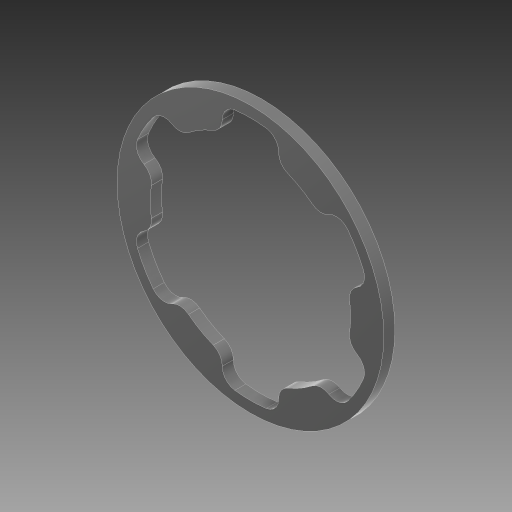
# Autodesk Inventor part: MAXSpline Spacers
Saved by Autodesk Inventor 2023 (Build 270158030, 158C)
## iProperties
Created: 2023-01-27
Part Number: MAXSpline Spacers
Material: Acetal Resin, Black
Document SubType Name: Modeling
Designer: Max Boord
Density: 1.425 g/cm^3
Appearance: Smooth - Black
Author: Max Boord
Mass: 17.9779 g
Surface Area: 108.837 cm^2
Volume: 12.6161 cm^3
Autodesk Inventor part; units mm, degrees
ref_plane "YZ Plane" through (0, 0, 0) normal (1, 0, 0) x (0, 1, 0)
ref_plane "XZ Plane" through (0, 0, 0) normal (0, 1, 0) x (-1, 0, 0)
ref_plane "XY Plane" through (0, 0, 0) normal (0, 0, 1) x (1, 0, 0)
sketch "MAXSpline Spacer Profile" plane through (0, 0, 0) normal (0, 0, 1) x (1, 0, 0)
  circle A0 centre (0, 0) radius 19.05
  arc A1 (15.22, 4.1356) -> (16.1399, 6.7328) centre (14.2452, 5.9424) ccw
  arc A2 (15.22, 4.1356) -> (14.1626, 2.0366) centre (16.1947, 2.3288) ccw
  arc A3 (14.1626, -2.0366) -> (14.1626, 2.0366) centre (0, 0) ccw
  arc A4 (14.1626, -2.0366) -> (15.22, -4.1356) centre (16.1947, -2.3288) ccw
  arc A5 (16.1399, -6.7328) -> (15.22, -4.1356) centre (14.2452, -5.9424) ccw
  arc A6 (13.9007, -10.6112) -> (16.1399, -6.7328) centre (0, 0) ccw
  arc A7 (11.1915, -11.1131) -> (13.9007, -10.6112) centre (12.2689, -9.3655) ccw
  arc A8 (11.1915, -11.1131) -> (8.845, -11.2469) centre (10.1141, -12.8607) ccw
  arc A9 (5.3176, -13.2835) -> (8.845, -11.2469) centre (0, 0) ccw
  arc A10 (5.3176, -13.2835) -> (4.0285, -15.2487) centre (6.0806, -15.1894) ccw
  arc A11 (2.2392, -17.344) -> (4.0285, -15.2487) centre (1.9763, -15.3079) ccw
  arc A12 (-2.2392, -17.344) -> (2.2392, -17.344) centre (0, 0) ccw
  arc A13 (-4.0285, -15.2487) -> (-2.2392, -17.344) centre (-1.9763, -15.3079) ccw
  arc A14 (-4.0285, -15.2487) -> (-5.3176, -13.2835) centre (-6.0806, -15.1894) ccw
  arc A15 (-8.845, -11.2469) -> (-5.3176, -13.2835) centre (0, 0) ccw
  arc A16 (-8.845, -11.2469) -> (-11.1915, -11.1131) centre (-10.1141, -12.8607) ccw
  arc A17 (-13.9007, -10.6112) -> (-11.1915, -11.1131) centre (-12.2689, -9.3655) ccw
  arc A18 (-16.1399, -6.7328) -> (-13.9007, -10.6112) centre (0, 0) ccw
  arc A19 (-15.22, -4.1356) -> (-16.1399, -6.7328) centre (-14.2452, -5.9424) ccw
  arc A20 (-15.22, -4.1356) -> (-14.1626, -2.0366) centre (-16.1947, -2.3288) ccw
  arc A21 (-14.1626, 2.0366) -> (-14.1626, -2.0366) centre (0, 0) ccw
  arc A22 (-14.1626, 2.0366) -> (-15.22, 4.1356) centre (-16.1947, 2.3288) ccw
  arc A23 (-16.1399, 6.7328) -> (-15.22, 4.1356) centre (-14.2452, 5.9424) ccw
  arc A24 (-13.9007, 10.6112) -> (-16.1399, 6.7328) centre (0, 0) ccw
  arc A25 (-11.1915, 11.1131) -> (-13.9007, 10.6112) centre (-12.2689, 9.3655) ccw
  arc A26 (-11.1915, 11.1131) -> (-8.845, 11.2469) centre (-10.1141, 12.8607) ccw
  arc A27 (-5.3176, 13.2835) -> (-8.845, 11.2469) centre (0, 0) ccw
  arc A28 (-5.3176, 13.2835) -> (-4.0285, 15.2487) centre (-6.0806, 15.1894) ccw
  arc A29 (-2.2392, 17.344) -> (-4.0285, 15.2487) centre (-1.9763, 15.3079) ccw
  arc A30 (2.2392, 17.344) -> (-2.2392, 17.344) centre (0, 0) ccw
  arc A31 (4.0285, 15.2487) -> (2.2392, 17.344) centre (1.9763, 15.3079) ccw
  arc A32 (4.0285, 15.2487) -> (5.3176, 13.2835) centre (6.0806, 15.1894) ccw
  arc A33 (8.845, 11.2469) -> (5.3176, 13.2835) centre (0, 0) ccw
  arc A34 (8.845, 11.2469) -> (11.1915, 11.1131) centre (10.1141, 12.8607) ccw
  arc A35 (13.9007, 10.6112) -> (11.1915, 11.1131) centre (12.2689, 9.3655) ccw
  arc A36 (16.1399, 6.7328) -> (13.9007, 10.6112) centre (0, 0) ccw
  arc A37 (17.4067, -2.0716) -> (17.4067, 2.0716) centre (0, 0) ccw
  arc A38 (15.7454, -1.8738) -> (17.4067, -2.0716) centre (16.5761, -1.9727) ccw
  arc A39 (15.7454, -1.8738) -> (15.7454, 1.8738) centre (0, 0) ccw
  arc A40 (17.4067, 2.0716) -> (15.7454, 1.8738) centre (16.5761, 1.9727) ccw
  arc A41 (10.4974, 14.0389) -> (6.9093, 16.1104) centre (0, 0) ccw
  arc A42 (9.4955, 12.699) -> (10.4974, 14.0389) centre (9.9964, 13.3689) ccw
  arc A43 (9.4955, 12.699) -> (6.2499, 14.5728) centre (0, 0) ccw
  arc A44 (6.9093, 16.1104) -> (6.2499, 14.5728) centre (6.5796, 15.3416) ccw
  arc A45 (-6.9093, 16.1104) -> (-10.4974, 14.0389) centre (0, 0) ccw
  arc A46 (-6.2499, 14.5728) -> (-6.9093, 16.1104) centre (-6.5796, 15.3416) ccw
  arc A47 (-6.2499, 14.5728) -> (-9.4955, 12.699) centre (0, 0) ccw
  arc A48 (-10.4974, 14.0389) -> (-9.4955, 12.699) centre (-9.9964, 13.3689) ccw
  arc A49 (-17.4067, 2.0716) -> (-17.4067, -2.0716) centre (0, 0) ccw
  arc A50 (-15.7454, 1.8738) -> (-17.4067, 2.0716) centre (-16.5761, 1.9727) ccw
  arc A51 (-15.7454, 1.8738) -> (-15.7454, -1.8738) centre (0, 0) ccw
  arc A52 (-17.4067, -2.0716) -> (-15.7454, -1.8738) centre (-16.5761, -1.9727) ccw
  arc A53 (-10.4974, -14.0389) -> (-6.9093, -16.1104) centre (0, 0) ccw
  arc A54 (-9.4955, -12.699) -> (-10.4974, -14.0389) centre (-9.9964, -13.3689) ccw
  arc A55 (-9.4955, -12.699) -> (-6.2499, -14.5728) centre (0, 0) ccw
  arc A56 (-6.9093, -16.1104) -> (-6.2499, -14.5728) centre (-6.5796, -15.3416) ccw
  arc A57 (6.9093, -16.1104) -> (10.4974, -14.0389) centre (0, 0) ccw
  arc A58 (6.2499, -14.5728) -> (6.9093, -16.1104) centre (6.5796, -15.3416) ccw
  arc A59 (6.2499, -14.5728) -> (9.4955, -12.699) centre (0, 0) ccw
  arc A60 (10.4974, -14.0389) -> (9.4955, -12.699) centre (9.9964, -13.3689) ccw
  dimension "d0" = 38.1
  measures "d0" diameter of A0
sketch "Sketch1" plane through (0, 0, 0) normal (0, 0, 1) x (1, 0, 0)
  circle A0 centre (0, 0) radius 19.05
  arc A1 (15.22, 4.1356) -> (16.1399, 6.7328) centre (14.2452, 5.9424) ccw
  arc A2 (15.22, 4.1356) -> (14.1626, 2.0366) centre (16.1947, 2.3288) ccw
  arc A3 (14.1626, -2.0366) -> (14.1626, 2.0366) centre (0, 0) ccw
  arc A4 (14.1626, -2.0366) -> (15.22, -4.1356) centre (16.1947, -2.3288) ccw
  arc A5 (16.1399, -6.7328) -> (15.22, -4.1356) centre (14.2452, -5.9424) ccw
  arc A6 (13.9007, -10.6112) -> (16.1399, -6.7328) centre (0, 0) ccw
  arc A7 (11.1915, -11.1131) -> (13.9007, -10.6112) centre (12.2689, -9.3655) ccw
  arc A8 (11.1915, -11.1131) -> (8.845, -11.2469) centre (10.1141, -12.8607) ccw
  arc A9 (5.3176, -13.2835) -> (8.845, -11.2469) centre (0, 0) ccw
  arc A10 (5.3176, -13.2835) -> (4.0285, -15.2487) centre (6.0806, -15.1894) ccw
  arc A11 (2.2392, -17.344) -> (4.0285, -15.2487) centre (1.9763, -15.3079) ccw
  arc A12 (-2.2392, -17.344) -> (2.2392, -17.344) centre (0, 0) ccw
  arc A13 (-4.0285, -15.2487) -> (-2.2392, -17.344) centre (-1.9763, -15.3079) ccw
  arc A14 (-4.0285, -15.2487) -> (-5.3176, -13.2835) centre (-6.0806, -15.1894) ccw
  arc A15 (-8.845, -11.2469) -> (-5.3176, -13.2835) centre (0, 0) ccw
  arc A16 (-8.845, -11.2469) -> (-11.1915, -11.1131) centre (-10.1141, -12.8607) ccw
  arc A17 (-13.9007, -10.6112) -> (-11.1915, -11.1131) centre (-12.2689, -9.3655) ccw
  arc A18 (-16.1399, -6.7328) -> (-13.9007, -10.6112) centre (0, 0) ccw
  arc A19 (-15.22, -4.1356) -> (-16.1399, -6.7328) centre (-14.2452, -5.9424) ccw
  arc A20 (-15.22, -4.1356) -> (-14.1626, -2.0366) centre (-16.1947, -2.3288) ccw
  arc A21 (-14.1626, 2.0366) -> (-14.1626, -2.0366) centre (0, 0) ccw
  arc A22 (-14.1626, 2.0366) -> (-15.22, 4.1356) centre (-16.1947, 2.3288) ccw
  arc A23 (-16.1399, 6.7328) -> (-15.22, 4.1356) centre (-14.2452, 5.9424) ccw
  arc A24 (-13.9007, 10.6112) -> (-16.1399, 6.7328) centre (0, 0) ccw
  arc A25 (-11.1915, 11.1131) -> (-13.9007, 10.6112) centre (-12.2689, 9.3655) ccw
  arc A26 (-11.1915, 11.1131) -> (-8.845, 11.2469) centre (-10.1141, 12.8607) ccw
  arc A27 (-5.3176, 13.2835) -> (-8.845, 11.2469) centre (0, 0) ccw
  arc A28 (-5.3176, 13.2835) -> (-4.0285, 15.2487) centre (-6.0806, 15.1894) ccw
  arc A29 (-2.2392, 17.344) -> (-4.0285, 15.2487) centre (-1.9763, 15.3079) ccw
  arc A30 (2.2392, 17.344) -> (-2.2392, 17.344) centre (0, 0) ccw
  arc A31 (4.0285, 15.2487) -> (2.2392, 17.344) centre (1.9763, 15.3079) ccw
  arc A32 (4.0285, 15.2487) -> (5.3176, 13.2835) centre (6.0806, 15.1894) ccw
  arc A33 (8.845, 11.2469) -> (5.3176, 13.2835) centre (0, 0) ccw
  arc A34 (8.845, 11.2469) -> (11.1915, 11.1131) centre (10.1141, 12.8607) ccw
  arc A35 (13.9007, 10.6112) -> (11.1915, 11.1131) centre (12.2689, 9.3655) ccw
  arc A36 (16.1399, 6.7328) -> (13.9007, 10.6112) centre (0, 0) ccw
  arc A37 (17.4067, -2.0716) -> (17.4067, 2.0716) centre (0, 0) ccw
  arc A38 (15.7454, -1.8738) -> (17.4067, -2.0716) centre (16.5761, -1.9727) ccw
  arc A39 (15.7454, -1.8738) -> (15.7454, 1.8738) centre (0, 0) ccw
  arc A40 (17.4067, 2.0716) -> (15.7454, 1.8738) centre (16.5761, 1.9727) ccw
  arc A41 (10.4974, 14.0389) -> (6.9093, 16.1104) centre (0, 0) ccw
  arc A42 (9.4955, 12.699) -> (10.4974, 14.0389) centre (9.9964, 13.3689) ccw
  arc A43 (9.4955, 12.699) -> (6.2499, 14.5728) centre (0, 0) ccw
  arc A44 (6.9093, 16.1104) -> (6.2499, 14.5728) centre (6.5796, 15.3416) ccw
  arc A45 (-6.9093, 16.1104) -> (-10.4974, 14.0389) centre (0, 0) ccw
  arc A46 (-6.2499, 14.5728) -> (-6.9093, 16.1104) centre (-6.5796, 15.3416) ccw
  arc A47 (-6.2499, 14.5728) -> (-9.4955, 12.699) centre (0, 0) ccw
  arc A48 (-10.4974, 14.0389) -> (-9.4955, 12.699) centre (-9.9964, 13.3689) ccw
  arc A49 (-17.4067, 2.0716) -> (-17.4067, -2.0716) centre (0, 0) ccw
  arc A50 (-15.7454, 1.8738) -> (-17.4067, 2.0716) centre (-16.5761, 1.9727) ccw
  arc A51 (-15.7454, 1.8738) -> (-15.7454, -1.8738) centre (0, 0) ccw
  arc A52 (-17.4067, -2.0716) -> (-15.7454, -1.8738) centre (-16.5761, -1.9727) ccw
  arc A53 (-10.4974, -14.0389) -> (-6.9093, -16.1104) centre (0, 0) ccw
  arc A54 (-9.4955, -12.699) -> (-10.4974, -14.0389) centre (-9.9964, -13.3689) ccw
  arc A55 (-9.4955, -12.699) -> (-6.2499, -14.5728) centre (0, 0) ccw
  arc A56 (-6.9093, -16.1104) -> (-6.2499, -14.5728) centre (-6.5796, -15.3416) ccw
  arc A57 (6.9093, -16.1104) -> (10.4974, -14.0389) centre (0, 0) ccw
  arc A58 (6.2499, -14.5728) -> (6.9093, -16.1104) centre (6.5796, -15.3416) ccw
  arc A59 (6.2499, -14.5728) -> (9.4955, -12.699) centre (0, 0) ccw
  arc A60 (10.4974, -14.0389) -> (9.4955, -12.699) centre (9.9964, -13.3689) ccw
  constraints: 1 other
extrude "Extrusion1" add sketch "Sketch1" along normal mid plane 1.5875 contours A0 | A38 A39 A40 A37 | A42 A43 A44 A41 | A46 A47 A48 A45 | A50 A51 A52 A49 | A54 A55 A56 A53 | A58 A59 A60 A57
extrude "Extrusion2" [suppressed]
fillet "Fillet1" [suppressed]
mirror "Mirror1" [suppressed]
body "Solid1"
